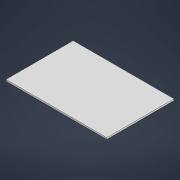
# Autodesk Inventor part: Base Plate
Saved by Autodesk Inventor 2022 (Build 260153000, 153)
## iProperties
Created: 2023-06-23
Part Number: Base Plate
Material: Generic
Document SubType Name: Modeling
Designer: Ryan Mitcham
Density: 1 g/cm^3
Appearance: Default
Author: Ryan Mitcham
Autodesk Inventor part; units mm, degrees
ref_plane "YZ Plane" through (0, 0, 0) normal (1, 0, 0) x (0, 1, 0)
ref_plane "XZ Plane" through (0, 0, 0) normal (0, 1, 0) x (-1, 0, 0)
ref_plane "XY Plane" through (0, 0, 0) normal (0, 0, 1) x (1, 0, 0)
sketch "Sketch1" plane through (0, 0, 0) normal (0, 1, 0) x (-1, 0, 0)
  line L0 (600, -400) -> (-600, -400)
  line L1 (-600, -400) -> (-600, 400)
  line L2 (-600, 400) -> (600, 400)
  line L3 (600, 400) -> (600, -400)
  point P0 (0, 0)
  point P1 (0, -400)
  point P2 (-600, 0)
  dimension "d0" = 1200
  dimension "d1" = 800
  constraints: 8 end point, 2 midpoint, 2 parallel, 1 horizontal, 1 horizontal alignment, 1 perpendicular, 1 vertical alignment
  measures "d0" distance of L0.start L0.end
  measures "d1" distance of L0.end L1.end
extrude "Extrusion1" add sketch "Sketch1" along normal blind 18
body "Solid1"
